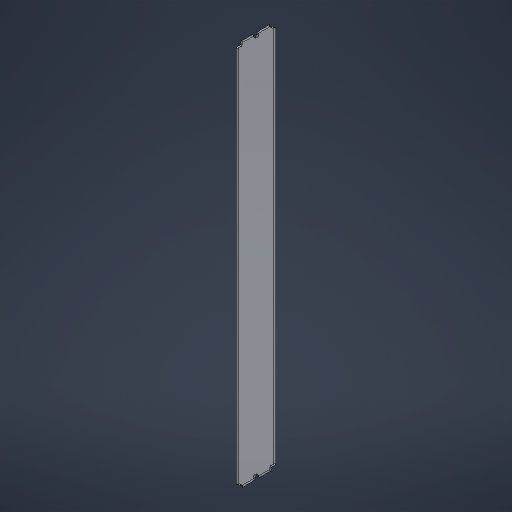
# Autodesk Inventor part: PLATE,TOP,BACK
Saved by Autodesk Inventor 2026 (Build 300175000, 175)
## iProperties
Created: 2026-02-18
Part Number: PLATE,TOP,BACK
Material: Polycarbonate, Clear
Document SubType Name: Modeling
Designer: littl
Density: 1.2 g/cm^3
Appearance: Polycarbonate - Clear
Author: littl
Autodesk Inventor part; units mm, degrees
ref_plane "YZ Plane" through (0, 0, 0) normal (1, 0, 0) x (0, 1, 0)
ref_plane "XZ Plane" through (0, 0, 0) normal (0, 1, 0) x (-1, 0, 0)
ref_plane "XY Plane" through (0, 0, 0) normal (0, 0, 1) x (1, 0, 0)
sketch "Sketch1" plane through (0, 0, 0) normal (1, 0, 0) x (0, 1, 0)
  line L0 (-323.85, -31.75) -> (323.85, -31.75)
  line L1 (323.85, -31.75) -> (323.85, 31.75)
  line L2 (323.85, 31.75) -> (-323.85, 31.75)
  line L3 (-323.85, 31.75) -> (-323.85, -31.75)
  line L4 (-323.85, -31.75) -> (323.85, 31.75) construction
  line L5 (323.85, -31.75) -> (-323.85, 31.75) construction
  line L6 (-323.85, 25.4) -> (-328.6125, 25.4)
  line L7 (-328.6125, 25.4) -> (-328.6125, -25.4)
  line L8 (-328.6125, -25.4) -> (-323.85, -25.4)
  line L9 (-323.85, -25.4) -> (-323.85, 25.4)
  line L10 (-328.6125, 3.175) -> (-323.85, 3.175)
  line L11 (-323.85, 3.175) -> (-323.85, -3.175)
  line L12 (-323.85, -3.175) -> (-328.6125, -3.175)
  line L13 (-328.6125, -3.175) -> (-328.6125, 3.175)
  line L14 (323.85, 25.4) -> (328.6125, 25.4)
  line L15 (328.6125, 25.4) -> (328.6125, -25.4)
  line L16 (328.6125, -25.4) -> (323.85, -25.4)
  line L17 (323.85, -25.4) -> (323.85, 25.4)
  line L18 (323.85, -3.175) -> (328.6125, -3.175)
  line L19 (328.6125, -3.175) -> (328.6125, 3.175)
  line L20 (328.6125, 3.175) -> (323.85, 3.175)
  line L21 (323.85, 3.175) -> (323.85, -3.175)
  point P0 (0, 0)
  point P1 (-328.6125, 0)
  point P2 (-326.2312, -3.175)
  point P3 (-326.2312, 3.175)
  point P4 (-323.85, 0)
  point P5 (328.6125, 0)
  point P6 (328.6125, 0)
  dimension "d0" = 647.7
  dimension "d1" = 63.5
  dimension "d2" = 50.8
  dimension "d3" = 4.7625
  dimension "d4" = 6.35
  dimension "d5" = 4.7625
  dimension "d6" = 50.8
  dimension "d7" = 6.35
  constraints: 44 end point, 10 parallel, 8 midpoint, 6 point on line, 5 horizontal, 5 perpendicular, 3 horizontal alignment, 1 coincident
  measures "d0" distance of L2.end L1.end
  measures "d1" distance of L1.end L0.end
  measures "d2" distance of L6.end L7.end
  measures "d3" distance of L6.start L6.end
  measures "d4" distance of point (-326.231, -3.175) point (-326.231, 3.175)
  measures "d5" distance of L15.end L16.end
  measures "d6" distance of L14.end L15.end
  measures "d7" distance between parallel lines of L20 L18
extrude "Extrusion1" add sketch "Sketch1" along normal blind 3.175 contours L3 L2 L1 L0 | L8 L7 L12 L3 | L1 L18 L15 L16 | L10 L7 L6 L3 | L1 L14 L15 L20
fillet "Fillet1" radius 1.5875 20 edges at (1.5875, 323.85, 31.75) (1.5875, 323.85, 25.4) (1.5875, 328.6125, 25.4) (1.5875, 323.85, -3.175) (1.5875, 323.85, 3.175) (1.5875, 328.6125, 3.175) (1.5875, 328.6125, -3.175) (1.5875, 328.6125, -25.4) (1.5875, 323.85, -25.4) (1.5875, 323.85, -31.75) (1.5875, -323.85, 31.75) (1.5875, -323.85, 25.4) (1.5875, -328.6125, 25.4) (1.5875, -328.6125, 3.175) (1.5875, -323.85, 3.175) (1.5875, -328.6125, -3.175) (1.5875, -323.85, -3.175) (1.5875, -328.6125, -25.4) (1.5875, -323.85, -25.4) (1.5875, -323.85, -31.75)
equation "\"d2\" = d6"
body "Solid1"
